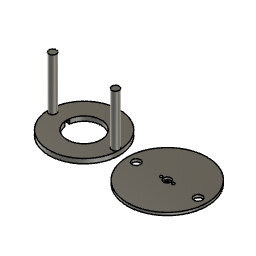
Lens Servo Coupling (Autodesk Fusion 360 design; units mm, degrees)
Autodesk Fusion 360 part; units mm, degrees
note: some values were not read from the file. Chosen so that the rebuilt part matches the saved one: which face or edge a step refers to; which pieces of a blend or face edit are solid.
sketch "Sketch1" plane through (0, 0, 0) normal (0, 0, 1) x (1, 0, 0)
  circle A0 centre (0, 0) radius 38
  circle A1 centre (0, 0) radius 20
  dimension "d1" = 76
  dimension "d2" = 40
  constraint coincident A0.centre A1.centre
  measures "d1" diameter of A0
  measures "d2" diameter of A1
extrude "Extrude1" add sketch "Sketch1" along normal blind 3 makes body 1
sketch "Sketch2" plane through (0, 0, 3) normal (0, 0, 1) x (-1, 0, 0)
  circle A0 centre (0, 0) radius 20
  circle A1 centre (0, 0) radius 38
sketch "Sketch3" plane through (0, 0, 3) normal (0, 0, 1) x (-1, 0, 0)
sketch "Sketch4" plane through (0, 0, 3) normal (0, 0, 1) x (-1, 0, 0)
  circle A0 centre (34, 0) radius 4
  circle A1 centre (-34, 0) radius 4
  line L0 (25, 0) -> (25, -2.5)
  line L1 (25, -2.5) -> (19.84, -2.5)
  line L2 (25, 0) -> (25, 2.5)
  line L3 (25, 2.5) -> (19.84, 2.5)
  circle A2 centre (0, 0) radius 20
  dimension "d6" = 2.5
  constraint perpendicular L0 L1
  constraint coincident A2.centre origin
  measures "d6" distance of L0.start L0.end
extrude "Extrude2" add sketch "Sketch2" against normal blind 5 contours A0 bodies 1
extrude "Extrude3" cut 1 faces at (-4.7423, 7.1112, -2) along direction (0, 0, 1) blind 35 on bodies 1 bodies 1
sketch "Sketch5" plane through (0, 0, 3) normal (0, 0, 1) x (-1, 0, 0)
  circle A0 centre (0, 0) radius 20
  circle A1 centre (0, 0) radius 38
extrude "Extrude4" cut sketch "Sketch4" against normal blind 28 contours L0 L1 L2 L3 A2 bodies 1
extrude "Extrude6" add sketch "Sketch4" along normal blind 51 contours A0 | A1 bodies 1
sketch "Sketch6" plane through (0, 0, 54) normal (0, 0, 1) x (-1, 0, 0)
  circle A0 centre (34, 0) radius 4
  circle A1 centre (0, 0) radius 38
  circle A2 centre (0, 0) radius 4
  line L0 (0, 0) -> (2, 0)
  line L1 (2, 0) -> (8, 0)
  circle A3 centre (8, 0) radius 1.5
  line L2 (0, 0) -> (0, 4)
  circle A4 centre (-8, 0) radius 1.5
  dimension "d17" = 8
  dimension "d18" = 3
  constraint coincident A1.centre A2.centre
  constraint tangent A0 A1
  constraint horizontal L0
  constraint parallel L0 L1
  constraint coincident L1.end A3.centre
  constraint coincident A2 L2.end
  constraint perpendicular L0 L2
  constraint symmetric A3 L2 A4
  measures "d17" diameter of A2
  measures "d18" diameter of A3
extrude "Extrude7" add sketch "Sketch6" along normal blind 5 separate body contours A0 | A1 makes body 2
sketch "Sketch7" plane through (0, 0, 0) normal (0, 0, 1) x (1, 0, 0)
  line L0 (0, 0) -> (-0.0025, 0)
  constraint coincident L0.start origin
  constraint horizontal L0
move_body "Move1" bodies 2 to x (1, 0, 0) y (0, 1, 0) z (0, 0, 1) at (-0.0025, 0, -59)
move_body "Move2" bodies 2 to x (1, 0, 0) y (0, 1, 0) z (0, 0, 1) at (90, 0, 0)
move_body "Move3" bodies 2 to x (1, 0, 0) y (0, 1, 0) z (0, 0, 1) at (0, 0, 5)
sketch "Sketch8" plane through (0, 0, 5) normal (0, 0, 1) x (-1, 0, 0)
  circle A0 centre (-97.9975, 0) radius 1.5
  circle A1 centre (-89.9975, 0) radius 4
  circle A2 centre (-81.9975, 0) radius 1.5
  circle A3 centre (-89.9975, 0) radius 38
  circle A4 centre (-89.9975, 0) radius 43
  dimension "d21" = 86
  constraint concentric A1 A4
  measures "d21" diameter of A4
extrude "Extrude8" add sketch "Sketch8" against normal blind 5 contours A4 bodies 2
sketch "Sketch9" plane through (0, 0, 5) normal (0, 0, 1) x (-1, 0, 0)
  circle A0 centre (-89.9975, 0) radius 43
  circle A1 centre (-97.9975, 0) radius 1.5
  circle A2 centre (-89.9975, 0) radius 4
  circle A3 centre (-81.9975, 0) radius 1.5
  circle A4 centre (-123.4975, 0) radius 4.5
  line L0 (-89.9975, 0) -> (-89.9975, -4)
  circle A5 centre (-56.4975, 0) radius 4.5
  dimension "d25" = 9
  constraint coincident A0.centre A2.centre
  constraint coincident A2 L0.end
  constraint vertical L0
  constraint symmetric A4 L0 A5
  measures "d25" diameter of A4
extrude "Extrude9" cut sketch "Sketch9" against normal blind 25 contours A4 | A5 bodies 2
sketch "Sketch10" plane through (0, 0, 0) normal (0, 0, -1) x (1, 0, 0)
  circle A0 centre (123.4975, 0) radius 4.5
  circle A1 centre (56.4975, 0) radius 4.5
  circle A2 centre (89.9975, 0) radius 43
  circle A3 centre (97.9975, 0) radius 1.5
  circle A4 centre (89.9975, 0) radius 4
  circle A5 centre (81.9975, 0) radius 1.5
  circle A6 centre (89.9975, 0) radius 2
  dimension "d28" = 4
  constraint concentric A2 A6
  measures "d28" diameter of A6
extrude "Extrude10" add sketch "Sketch10" against normal blind 2 contours A4 bodies 2
extrude "Extrude11" add sketch "Sketch4" against normal blind 1 contours L0 L1 L2 L3 A2 bodies 1
extrude "Extrude12" add 1 faces at (-25.834, -9.0451, 0) along direction (0, 0, -1) blind 2 on bodies 1 bodies 1
move_body "Move4" bodies 1 to x (1, 0, 0) y (0, 1, 0) z (0, 0, 1) at (0, 0, 2)
extrude "Extrude13" add 2 faces at (35.1017, -0.7511, 56) (-33.1165, 0.6023, 56) along direction (0, 0, 1) blind 5 on bodies 1 bodies 1
extrude "Extrude14" cut 1 faces at (86.6791, -0.1987, 2) along direction (0, 0, -1) blind 1.5 on bodies 2 bodies 2
sketch "Sketch11" plane through (0, 0, 5) normal (0, 0, 1) x (-1, 0, 0)
  circle A0 centre (-123.4975, 0) radius 4.5
  circle A1 centre (-56.4975, 0) radius 4.5
  circle A2 centre (-89.9975, 0) radius 43
  circle A3 centre (-97.9975, 0) radius 1.5
  circle A4 centre (-89.9975, 0) radius 4
  circle A5 centre (-81.9975, 0) radius 1.5
  circle A6 centre (-97.9975, 0) radius 1.5
  circle A7 centre (-81.9975, 0) radius 1.5
  line L0 (-89.9975, 0) -> (-84.9975, 0)
  dimension "d39" = 5
  constraint concentric A3 A6
  constraint concentric A5 A7
  constraint coincident A2.centre A4.centre
  constraint horizontal L0
  measures "d39" distance of A2.centre L0.end
extrude "Extrude15" add sketch "Sketch11" against normal blind 5 contours A3 A6 | A5 A7 bodies 2
sketch "Sketch12" plane through (0, 0, 5) normal (0, 0, 1) x (-1, 0, 0)
  circle A0 centre (-123.4975, 0) radius 4.5
  circle A1 centre (-56.4975, 0) radius 4.5
  circle A2 centre (-89.9975, 0) radius 43
  circle A3 centre (-89.9975, 0) radius 4
  circle A4 centre (-83.4975, 0) radius 1.5
  dimension "d43" = 3
  measures "d43" diameter of A4
sketch "Sketch13" plane through (0, 0, 5) normal (0, 0, 1) x (1, 0, 0)
  circle A0 centre (96.5, 0) radius 1.5
  dimension "d45" = 3
  measures "d45" diameter of A0
extrude "Extrude16" cut sketch "Sketch12" sketch "Sketch13" against normal blind 5 contours A4 of sketch 2 bodies 2
extrude "Extrude17" cut 3 faces at (66.3083, 11.3334, 5) (81.0031, 0.0745, 5) (98.488, -0.1491, 5) along direction (0, 0, -1) blind 2 on bodies 2 bodies 2
extrude "Extrude18" add 2 faces at (-25, 0.8333, 1.3333) (-25, -0.8333, 3.3333) along direction (1, 0, 0) blind 1 on bodies 1 bodies 1
move_face "OffsetFaces1" offset 1.5 3 faces at (-19.6967, 3.4698, 0.6667) (-19.5029, -4.4313, 3.6667) (-19.9051, -1.9465, 4.6667) on bodies 1
sketch "Sketch14" plane through (0, 0, 5) normal (0, 0, 1) x (-1, 0, 0)
  circle A0 centre (0, 0) radius 18.5
  arc A1 (-38, 0) -> (38, 0) centre (0, 0) ccw
  circle A2 centre (34, 0) radius 4
  arc A3 (38, 0) -> (-38, 0) centre (0, 0) ccw
  circle A4 centre (-34, 0) radius 4
  line L0 (10, -65) -> (2, -65)
  line L1 (2, -65) -> (2, -57)
  line L2 (2, -57) -> (10, -57)
  line L3 (10, -57) -> (10, -65)
  dimension "d53" = 8
  dimension "d54" = 8
  constraint horizontal L0
  constraint vertical L1
  constraint horizontal L2
  constraint vertical L3
  measures "d53" distance of L0.start L0.end
  measures "d54" distance of L0.start L2.end
